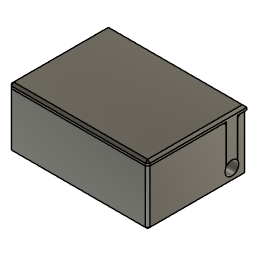
desky-esp32-box v5 (Autodesk Fusion 360 design; units mm, degrees)
Autodesk Fusion 360 part; units mm, degrees
sketch "Sketch1" plane through (0, 0, 0) normal (0, 0, 1) x (1, 0, 0)
  line L0 (0, 0) -> (56, 0)
  line L1 (56, 0) -> (56, 29)
  line L2 (56, 29) -> (0, 29)
  line L3 (0, 29) -> (0, 0)
  line L4 (0, 14.5) -> (56, 14.5) construction
  line L5 (0, 1.45) -> (56, 1.45)
  line L6 (0, 2.3) -> (56, 2.3)
  line L7 (0, 3.3) -> (56, 3.3)
  line L8 (0, 0.45) -> (56, 0.45)
  line L9 (0, 28.55) -> (56, 28.55)
  line L10 (0, 27.55) -> (56, 27.55)
  line L11 (0, 26.7) -> (56, 26.7)
  line L12 (0, 25.7) -> (56, 25.7)
  line L13 (56, 30) -> (0, 30)
  line L14 (56, 29) -> (0, 29)
  line L15 (0, 29) -> (0, 39)
  line L16 (0, 39) -> (56, 39)
  line L17 (56, 39) -> (56, 29)
  line L18 (-2, 29) -> (-2, 41)
  line L19 (-2, 41) -> (58, 41)
  line L20 (58, 41) -> (58, 29)
  line L21 (58, -2) -> (58, 29)
  line L22 (-2, -2) -> (58, -2)
  line L23 (-2, 29) -> (-2, -2)
  line L24 (28, 41) -> (28, -2) construction
  dimension "d1" = 56
  dimension "d2" = 29
  dimension "d3" = 13.05
  dimension "d4" = 12.2
  dimension "d5" = 11.2
  dimension "d6" = 14.05
  dimension "d7" = 1
  dimension "d8" = 10
  dimension "d9" = 2
  constraint horizontal L0
  constraint vertical L1
  constraint horizontal L2
  constraint vertical L3
  constraint coincident L0.start L3.end
  constraint midpoint L3 L4.start
  constraint midpoint L1 L4.end
  constraint symmetric L4 L5.start L10.start
  constraint symmetric L4 L5.end L10.end
  constraint symmetric L4 L6.start L11.start
  constraint symmetric L4 L6.end L11.end
  constraint symmetric L4 L7.start L12.start
  constraint symmetric L4 L7.end L12.end
  constraint symmetric L4 L8.start L9.start
  constraint symmetric L4 L8.end L9.end
  constraint horizontal L14
  constraint vertical L15
  constraint horizontal L16
  constraint vertical L17
  constraint midpoint L19 L24.start
  constraint midpoint L22 L24.end
  measures "d1" distance of L0.start L0.end
  measures "d2" distance of L0.end L1.end
  measures "d8" distance of L2.end L15.end
extrude "Extrude1" add sketch "Sketch1" along normal blind 9 contours L0 L1 L3 L8 | L1 L3 L5 L8 | L1 L3 L6 L7 | L1 L3 L11 L12 | L1 L3 L9 L10 | L1 L2 L3 L9 L14 makes body 1 at (18.6667, 0, 3) makes body 2 at (18.6667, 26.7, 3) makes body 3 at (18.6667, 3.3, 3) makes body 4 at (18.6667, 27.55, 3)
extrude "Extrude2" add sketch "Sketch1" along normal blind 2 contours L0 L1 L3 L8 | L1 L3 L5 L6 | L1 L3 L7 L12 | L1 L3 L10 L11 | L1 L2 L3 L9 L14 | L13 L15 L16 L17 bodies 1 2 3 4 makes body 5 at (18.6667, 36, 0)
extrude "Extrude3" add sketch "Sketch1" along normal blind 24 bodies 1 5
extrude "Extrude4" add sketch "Sketch1" along normal blind 14 contours L2 L13 L14 L15 L17 bodies 1
ref_plane "WorkPlane1" through (28, 14.5, 12.35) normal (0, 0, 1) x (1, 0, 0)
sketch "Sketch2" plane through (0, 0, 0) normal (1, 0, 0) x (0, 1, 0)
  line L0 (29, 9) -> (29, 14)
  line L1 (29, 14) -> (30, 14)
  line L2 (30, 14) -> (30, 2)
  line L3 (30, 2) -> (39, 2)
  line L4 (39, 2) -> (39, 24)
  line L5 (39, 24) -> (0, 24)
  line L6 (0, 24) -> (0, 9)
  line L7 (0, 9) -> (1.45, 9)
  line L8 (1.45, 9) -> (1.45, 2)
  line L9 (1.45, 2) -> (2.3, 2)
  line L10 (2.3, 2) -> (2.3, 9)
  line L11 (2.3, 9) -> (3.3, 9)
  line L12 (3.3, 9) -> (3.3, 2)
  line L13 (3.3, 2) -> (25.7, 2)
  line L14 (25.7, 2) -> (25.7, 9)
  line L15 (25.7, 9) -> (26.7, 9)
  line L16 (26.7, 9) -> (26.7, 2)
  line L17 (26.7, 2) -> (27.55, 2)
  line L18 (27.55, 2) -> (27.55, 9)
  line L19 (27.55, 9) -> (29, 9)
  line L20 (0, 9) -> (0, 24)
  line L21 (0, 24) -> (39, 24)
  line L22 (29, 9) -> (29, 14)
  line L23 (25.7, 2) -> (3.3, 2)
  line L24 (25.7, 2) -> (25.7, 9)
  line L25 (26.7, 9) -> (25.7, 9)
  line L26 (29, 9) -> (27.55, 9)
  line L27 (1.45, 9) -> (0, 9)
  line L28 (3.3, 9) -> (2.3, 9)
  line L29 (27.94, 12.35) -> (1.06, 12.35)
  line L30 (3.3, 9) -> (25.7, 9) construction
  line L31 (14.5, 9) -> (14.5, 16.9) construction
  line L32 (14.5, 12.35) -> (10.5, 12.35) construction
  line L33 (10.5, 12.35) -> (10.5, 16.5)
  line L34 (10.5, 12.35) -> (10.5, 11.5)
  line L35 (10.5, 16.5) -> (14.5, 16.5)
  line L36 (10.5, 11.5) -> (14.5, 11.5)
  line L37 (18.5, 11.5) -> (14.5, 11.5)
  line L38 (18.5, 12.35) -> (18.5, 16.5)
  line L39 (18.5, 12.35) -> (18.5, 11.5)
  line L40 (18.5, 16.5) -> (14.5, 16.5)
  line L41 (39, 2) -> (39, 24)
  line L42 (30, 14) -> (30, 2)
  line L43 (30, 2) -> (39, 2)
  line L44 (39, 2) -> (39, 24)
  line L45 (39, 24) -> (30, 24)
  line L46 (30, 24) -> (30, 2)
  line L47 (34.5, 2) -> (34.5, 24) construction
  circle A0 centre (34.5, 5.5) radius 3
  line L48 (37, 2) -> (37, 24)
  line L49 (32, 2) -> (32, 24)
  circle A1 centre (34.5, 5.5) radius 4
  line L50 (34.5, 9.5) -> (30, 9.5)
  line L51 (34.5, 9.5) -> (39, 9.5)
  point P0 (34.5, 5.5)
  point P1 (34.5, 9.5)
  dimension "d19" = 4
  dimension "d20" = 4.15
  dimension "d21" = 0.85
  dimension "d24" = 3.5
  dimension "d25" = 6
  dimension "d26" = 2.5
  dimension "d53" = 1
  constraint coincident L11.end L12.start
  constraint coincident L14.end L15.start
  constraint midpoint L30 L31.start
  constraint perpendicular L29 L31
  constraint midpoint L29 L32.start
  constraint coincident L29 L32.end
  constraint perpendicular L31 L32
  constraint perpendicular L29 L33
  constraint perpendicular L29 L34
  constraint perpendicular L31 L35
  constraint coincident L31 L35.end
  constraint coincident L31 L36.end
  constraint perpendicular L31 L36
  constraint symmetric L31 L32.end L38.start
  constraint symmetric L31 L33.end L38.end
  constraint symmetric L31 L34.end L37.start
  constraint symmetric L31 L35.end L40.end
  constraint symmetric L31 L36.end L37.end
  constraint horizontal L43
  constraint vertical L44
  constraint horizontal L45
  constraint vertical L46
  constraint coincident L4.end L5.start
  constraint coincident L2.end L3.start
  constraint midpoint L43 L47.start
  constraint midpoint L45 L47.end
  constraint coincident L47 P0
  constraint coincident P0 A0.centre
  constraint symmetric L47 L48.start L49.start
  constraint symmetric L47 L48.end L49.end
  constraint coincident A1 P1
  constraint coincident L47 P1
  constraint coincident P1 L50.start
  constraint coincident L46 L50.end
  constraint symmetric L47 P1 L50.start
  constraint symmetric L47 L50.end L51.end
  measures "d19" distance of L32.start L32.end
  measures "d20" distance of L32.end L33.end
  measures "d21" distance of L32.end L34.end
  measures "d24" distance of L47.start P0
  measures "d25" diameter of A0
extrude "Extrude5" cut sketch "Sketch2" against normal blind 2 contours L29 L34 L36 L37 L39 | L29 L33 L35 L38 L40 bodies 1
ref_plane "WorkPlane2" through (28, 19.5, 0) normal (-1, 0, 0) x (0, -1, 0)
extrude "Extrude6" cut sketch "Sketch2" against normal blind 2 contours A0 L49 | A0 L48 L49 | A0 L48 bodies 1
extrude "Extrude7" add sketch "Sketch2" against normal blind 2 separate body contours L49 A1 L50 | L5 L21 L45 L48 L49 L50 L51 | A0 L48 L49 A1 | L48 A1 L51 makes body 6
mirror "Mirror1" about plane through (28, 19.5, 0) normal (-1, 0, 0) of "Extrude6"
mirror "Mirror2" about plane through (28, 19.5, 0) normal (-1, 0, 0) of "Extrude7" makes body 7
ref_plane "WorkPlane3" through (28, 19.5, 24) normal (0, 0, 1) x (1, 0, 0)
sketch "Sketch3" plane through (28, 19.5, 24) normal (0, 0, 1) x (1, 0, 0)
  line L0 (-30, -21.5) -> (30, -21.5)
  line L1 (30, -21.5) -> (30, 9.5)
  line L2 (30, 21.5) -> (30, 9.5)
  line L3 (-30, 21.5) -> (30, 21.5)
  line L4 (-28, 19.5) -> (28, 19.5)
  line L5 (28, -19.5) -> (28, 9.5)
  line L6 (28, 19.5) -> (28, 9.5)
  line L7 (-30, 9.5) -> (-30, 21.5)
  line L8 (-28, 9.5) -> (-28, 19.5)
  line L9 (-30, 9.5) -> (-30, -21.5)
  line L10 (-28, 9.5) -> (-28, -19.5)
  line L11 (-28, -19.5) -> (28, -19.5)
  line L12 (-27.86, 9.5) -> (-27.86, 19.36)
  line L13 (-27.86, 19.36) -> (27.86, 19.36)
  line L14 (27.86, 19.36) -> (27.86, 9.5)
  line L15 (27.86, -19.36) -> (27.86, 9.5)
  line L16 (-27.86, -19.36) -> (27.86, -19.36)
  line L17 (-27.86, 9.5) -> (-27.86, -19.36)
  line L18 (-25.5, 9.5) -> (-25.5, 17)
  line L19 (-25.5, 17) -> (25.5, 17)
  line L20 (25.5, 17) -> (25.5, 9.5)
  line L21 (25.5, -17) -> (25.5, 9.5)
  line L22 (-25.5, -17) -> (25.5, -17)
  line L23 (-25.5, 9.5) -> (-25.5, -17)
  dimension "d37" = 0.14
  dimension "d64" = 2.5
extrude "Extrude8" add sketch "Sketch3" against normal blind 2 separate body contours L12 L13 L14 L15 L16 L17 makes body 8
extrude "Extrude9" add sketch "Sketch3" along normal blind 2 contours L0 L1 L2 L3 L7 L9 | L4 L5 L6 L8 L10 L11 | L12 L13 L14 L15 L16 L17 | L18 L19 L20 L21 L22 L23 bodies 8
sketch "Sketch4" plane through (0, 37, 0) normal (0, 1, 0) x (-1, 0, 0)
  line L0 (0, 24) -> (0, 7.1583)
  line L1 (0, 7.1583) -> (2, 7.1583)
  line L2 (2, 7.1583) -> (2, 24)
  line L3 (2, 24) -> (0, 24)
move_face "OffsetFaces1" offset -0.1 1 faces at (-0.6667, 32, 12.7722) on bodies 6
extrude "Extrude10" cut sketch "Sketch4" against normal blind 0.1 bodies 6
move_face "OffsetFaces2" offset -0.1 1 faces at (56.6667, 37, 12.7722) on bodies 7
move_face "OffsetFaces3" offset -0.1 1 faces at (56.6667, 32, 12.7722) on bodies 7
combine "Combine1" operation add target body 8 tool bodies 7 6
extrude "Extrude11" cut sketch "Sketch2" against normal blind 2 contours L49 A1 L50 | L5 L21 L45 L48 L49 L50 L51 | A0 L48 L49 A1 | L48 A1 L51 bodies 1
mirror "Mirror3" about plane through (28, 19.5, 0) normal (-1, 0, 0) of "Extrude11"
chamfer "Chamfer1" distance 1 angle 45 15 edges at (58, -2, 12) (58, 19.5, 0) (28, -2, 0) (58, 41, 12) (28, 41, 0) (-2, 41, 12) (-2, 19.5, 0) (-2, -2, 12) (58, -2, 25) (28, -2, 26) (58, 19.5, 26) (28, 41, 26) (-2, 41, 25) (-2, 19.5, 26) (-2, -2, 25) on bodies 1 8
chamfer "Chamfer2" distance 1 angle 45 4 edges at (-2, 18.5, 14) (-2, 14.5, 16.5) (-2, 14.5, 11.5) (-2, 10.5, 14) on bodies 1
extrude "Extrude12" add sketch "Sketch2" along normal blind 4 contours L2 L3 L42 L43 L46 L49 A1 L50 | L3 L43 L49 A1 | A0 L49 A1 | L3 L43 A0 L48 L49 A1 | L3 L43 A1 | A0 L48 A1 | L3 L4 L41 L43 L44 L48 A1 L51 | L3 L43 L48 A1 bodies 1
chamfer "Chamfer3" distance 1 angle 45 2 edges at (2, 37, 9.5) (2, 32, 9.5) on bodies 1
chamfer "Chamfer3" distance 1 angle 45 2 edges at (4, 38, 9.5) (4, 31, 9.5) on bodies 1
mirror "Mirror4" about plane through (28, 19.5, 0) normal (-1, 0, 0) of "Extrude12", "Chamfer3"
chamfer "Chamfer4" distance 0.5 angle 45 4 edges at (28, 27.55, 9) (28, 26.7, 9) (28, 1.45, 9) (28, 2.3, 9) on bodies 1
fillet "Fillet1" radius 4 2 edges at (28, 25.7, 2) (28, 3.3, 2) on bodies 1
chamfer "Chamfer5" distance 1 angle 45 4 edges at (57, 32, 24) (57, 37, 24) (-1, 37, 24) (-1, 32, 24) on bodies 1
chamfer "Chamfer6" distance 1 angle 45 4 edges at (2.5, 19.5, 22) (28, 2.5, 22) (28, 36.5, 22) (53.5, 19.5, 22) on bodies 8
equation "d3 = ( 26.1 / 2 ) * 1 mm"
equation "d4 = ( 26.1 / 2 ) * 1 mm - 0.7 mm - 0.15 mm"
equation "d5 = ( 26.1 / 2 ) * 1 mm - 0.7 mm - 1 mm - 0.15 mm"
equation "d6 = ( 26.1 / 2 ) * 1 mm + 1 mm"
equation "d10 = 2 mm + 7 mm"
equation "d14 = 2 mm + 20 mm + 2 mm"
equation "d18 = 10.5 mm - 0.15 mm"
equation "d19 = ( 8 / 2 ) * 1 mm"
equation "d26 = ( 5 / 2 ) * 1 mm"
named bodies: "desky-esp32-base", "desky-esp32-cover"
